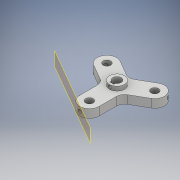
# Autodesk Inventor part: carrier2
Saved by Autodesk Inventor 2019 (Build 230136000, 136)
## iProperties
Created: 2019-12-31
Part Number: carrier2
Material: 一般
Document SubType Name: Modeling
Designer: louis
Density: 1 g/cm^3
Appearance: 預設
Author: louis
Autodesk Inventor part; units mm, degrees
sketch "草圖1" plane through (0, 0, 0) normal (0, 0, 1) x (1, 0, 0)
  line L0 (0, 0) -> (-28.5788, 16.5) construction
  line L1 (0, 0) -> (0, -33) construction
  circle A0 centre (28.5788, 16.5) radius 4.5
  circle A1 centre (0, -33) radius 4.5
  circle A2 centre (-28.5788, 16.5) radius 4.5
  line L2 (-22.8288, 26.4593) -> (-5.0753, 16.2093)
  arc A3 (-5.0753, 16.2093) -> (5.0753, 16.2093) centre (0, 25) ccw
  line L3 (5.0753, 16.2093) -> (22.8288, 26.4593)
  line L4 (22.8288, 26.4593) -> (22.8288, 26.4593)
  arc A4 (34.3288, 6.5407) -> (22.8288, 26.4593) centre (28.5788, 16.5) ccw
  line L5 (34.3288, 6.5407) -> (16.5753, -3.7093)
  arc A5 (16.5753, -3.7093) -> (11.5, -12.5) centre (21.6506, -12.5) ccw
  line L6 (11.5, -12.5) -> (11.5, -33)
  arc A6 (-11.5, -33) -> (11.5, -33) centre (0, -33) ccw
  line L7 (-11.5, -33) -> (-11.5, -12.5)
  arc A7 (-11.5, -12.5) -> (-16.5753, -3.7093) centre (-21.6506, -12.5) ccw
  line L8 (-16.5753, -3.7093) -> (-34.3288, 6.5407)
  arc A8 (-22.8288, 26.4593) -> (-34.3288, 6.5407) centre (-28.5788, 16.5) ccw
  line L9 (0, 0) -> (28.5788, 16.5) construction
  dimension "d0" = 33
  dimension "d4" = 120
  dimension "d5" = 33
  dimension "d6" = 9
  dimension "d9" = 7
  dimension "d10" = 7
  dimension "d11" = 7
  dimension "d12" = 33
  dimension "d13" = 120
  dimension "d35" = 25
  constraints: 20 end point, 12 point on circle, 12 tangent, 9 centre point, 4 equal length, 4 parallel, 3 concentric, 2 coincident, 2 equal radius, 1 vertical
  measures "d0" distance of L0.start L0.end
  measures "d5" distance of L0.start L1.end
  measures "d6" diameter of A2
  measures "d9" radial gap between concentric circles of A8 A2
  measures "d10" radial gap between concentric circles of A4 A0
  measures "d11" radial gap between concentric circles of A6 A1
  measures "d12" distance of L0.start L9.end
  measures "d35" distance of L0.start A3.centre
extrude "擠出1" add sketch "草圖1" along normal blind 10
ref_plane "工作平面1" through (0, -44.5, 0) normal (0, 1, 0) x (-1, 0, 0)
ref_plane "工作平面2" through (40.0788, 16.5, 0) normal (1, 0, 0) x (0, 1, 0)
ref_plane "工作平面3" through (-34.3288, 26.4593, 0) normal (-0.5, 0.8660254, 0) x (-0.8660254, -0.5, 0)
sketch "草圖2" plane through (-34.3288, 26.4593, 0) normal (-0.5, 0.8660254, 0) x (-0.8660254, -0.5, 0)
  point P0 (-16.5, 0)
  point P1 (0.7704, 4.0178)
hole "孔1" [suppressed]
sketch "草圖3" plane through (0, 0, 10) normal (0, 0, 1) x (1, 0, 0)
  circle A0 centre (0, 0) radius 5
  circle A1 centre (0, 0) radius 9
  line L0 (2.5, -4.3301) -> (2.5, -6.3301)
  line L1 (2.5, -6.3301) -> (-2.5, -6.3301)
  line L2 (-2.5, -6.3301) -> (-2.5, -4.3301)
  line L3 (0, -5) -> (0, -7)
  dimension "d48" = 10
  dimension "d49" = 18
  dimension "d50" = 5
  dimension "d51" = 2
  dimension "d52" = 2
  constraints: 8 end point, 3 point on circle, 2 centre point, 2 coincident, 2 perpendicular, 2 vertical, 1 parallel, 1 other
  measures "d48" diameter of A0
  measures "d49" diameter of A1
  measures "d50" distance of L0.end L1.end
  measures "d51" distance of L0.start L0.end
  measures "d52" distance of L3.start L3.end
extrude "擠出2" add sketch "草圖3" along normal blind 5
sketch "草圖4" plane through (0, 0, 10) normal (0, 0, 1) x (1, 0, 0)
  arc A0 (2.5, -4.3301) -> (-2.5, -4.3301) centre (0, 0) ccw projected
  line L0 (2.5, -4.3301) -> (2.5, -6.3301) projected
  line L1 (2.5, -6.3301) -> (-2.5, -6.3301) projected
  line L2 (-2.5, -6.3301) -> (-2.5, -4.3301) projected
  circle A1 centre (0, 0) radius 9 projected
extrude "擠出3" cut sketch "草圖4" against normal blind 10 contours L0 L1 L2 A0
ref_plane "工作平面4" through (0, -9, 10) normal (0, 1, 0) x (-1, 0, 0)
sketch "草圖5" plane through (0, -9, 10) normal (0, 1, 0) x (-1, 0, 0)
  point P0 (0, -10)
  point P1 (-0.3363, 2.4073)
hole "孔2" at (0.3363, -9, 12.4073) direction (0, 1, 0) diameter 3.242 end up to surface countersink diameter 4 countersink angle 90 thread size "M4x0.7" class "6H" standard "ISO Metric profile"
ref_plane "工作平面5" through (-5.75, -42.9593, 0) normal (-0.5, -0.8660254, 0) x (0.8660254, -0.5, 0)
ref_plane "工作平面6" through (0, -44.5, 0) normal (0, 1, 0) x (-1, 0, 0)
sketch "草圖6" plane through (0, -44.5, 0) normal (0, 1, 0) x (-1, 0, 0)
  line L0 (-11.5, 0) -> (11.5, 0) projected
  line L1 (-11.5, 0) -> (-11.5, 10) projected
  line L2 (11.5, 10) -> (-11.5, 10) projected
  line L3 (11.5, 0) -> (11.5, 10) projected
  circle A0 centre (0, 5) radius 2
  point P0 (0, 0)
  dimension "d64" = 4
  dimension "d65" = 5
  constraints: 1 centre point
  measures "d64" diameter of A0
  measures "d65" distance from line of L0 A0.centre
extrude "擠出4" cut sketch "草圖6" along normal up to next contours A0
pattern_circular "環形陣列2" count 3 over 360 about axis through (0, 0, -10) along (0, 0, 1) of "擠出4"
thread "螺紋1" size "M4x0.7" class "6H" standard "ANSI Metric M Profile" full length
thread "螺紋2" size "M4x0.7" class "6H" standard "ANSI Metric M Profile" full length
thread "螺紋3" size "M4x0.7" class "6H" standard "ANSI Metric M Profile" full length
equation "\"d0\" = d5"
equation "\"d10\" = d9"
equation "\"d11\" = d9"
equation "\"d12\" = d5"
